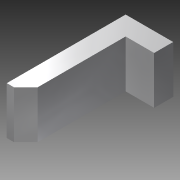
# Autodesk Inventor part: Robot-Clamp
Saved by Autodesk Inventor 2015 (Build 190159000, 159)
## iProperties
Shininess: 21.0
Length Units: 11269
Angle Units: 11279
Time Units: 11290
Mass Units: 11283
Length Display Precision: 3
Angle Display Precision: 2
Created: 2001-08-22
Part Number: Robot-Clamp
Document SubType Name: ﾓﾃﾞﾘﾝｸﾞ
Designer: Administrator
Density: 1 g/cm^3
Material: Generic
Appearance: Chrome - Polished
Density: 0.0
Volumn: 0.0
Area: 0.0
PropertySet Name: Model Information
Control State: 0
Master: False
Checked Out: False
Author: Administrator
Autodesk Inventor part; units mm, degrees
ref_plane "YZ Plane" through (0, 0, 0) normal (1, 0, 0) x (0, 1, 0)
ref_plane "XZ Plane" through (0, 0, 0) normal (0, 1, 0) x (-1, 0, 0)
ref_plane "XY Plane" through (0, 0, 0) normal (0, 0, 1) x (1, 0, 0)
sketch "ｽｹｯﾁ1" plane through (0, 0, 0) normal (0, 0, 1) x (1, 0, 0)
  line L0 (-1.8494, 20) -> (18.1506, 20)
  line L1 (18.1506, 20) -> (18.1506, 12)
  line L2 (18.1506, 12) -> (-1.8494, 12)
  line L3 (-1.8494, 12) -> (-1.8494, 20)
  line L4 (-1.8494, 20) -> (6.1506, 20)
  line L5 (6.1506, 20) -> (6.1506, -25)
  line L6 (1.1506, -30) -> (-1.8494, -30)
  line L7 (-1.8494, -30) -> (-1.8494, 20)
  line L8 (6.1506, -25) -> (1.1506, -30)
  point P0 (6.1506, -30)
  dimension "d0" = 20
  dimension "d1" = 8
  dimension "d2" = 50
  dimension "d3" = 5
  dimension "d4" = 5
  dimension "d5" = 8
  constraints: 18 end point, 4 parallel, 2 horizontal, 2 perpendicular, 2 point on line
  measures "d0" distance of L0.start L0.end
  measures "d1" distance of L0.end L1.end
  measures "d2" distance of L6.end L0.start
  measures "d3" distance of L5.end point (6.151, -30)
  measures "d4" distance of L6.start point (6.151, -30)
  measures "d5" distance between parallel lines of L7 L5
extrude "Extrusion1" add sketch "ｽｹｯﾁ1" along normal blind 20
equation "\"d4\" = d3"
body "Solid1"
